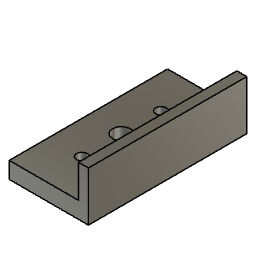
전방 덮개 브라켓 (Autodesk Fusion 360 design; units mm, degrees)
Autodesk Fusion 360 part; units mm, degrees
sketch "스케치1" plane through (0, 0, 0) normal (0, 0, 1) x (1, 0, 0)
  line L0 (10, 24) -> (-10, 24)
  line L1 (-10, 24) -> (-10, -24)
  line L2 (-10, -24) -> (10, -24)
  line L3 (10, -24) -> (10, 24)
  line L4 (10, 24) -> (-10, -24) construction
  line L5 (-10, 24) -> (10, -24) construction
  circle A0 centre (0, 0) radius 2.65
  line L6 (0, 0) -> (0, 12)
  circle A1 centre (0, 12) radius 1.6
  line L7 (0, 0) -> (0, -12)
  circle A2 centre (0, -12) radius 1.6
  line L8 (10, 24) -> (11, 24)
  line L9 (11, 24) -> (11, -24)
  line L10 (11, -24) -> (10, -24)
  line L11 (10, -24) -> (10, 24)
  line L12 (11, 24) -> (14, 24)
  line L13 (14, 24) -> (14, -24)
  line L14 (14, -24) -> (11, -24)
  line L15 (11, -24) -> (11, 24)
  line L16 (10, -6) -> (14, -6)
  dimension "d1" = 20
  dimension "d2" = 48
  dimension "d3" = 5.3
  dimension "d4" = 12
  dimension "d5" = 3.2
  dimension "d6" = 12
  dimension "d7" = 3.2
  dimension "d12" = 3
  constraint horizontal L0
  constraint perpendicular L0 L1
  constraint parallel L0 L2
  constraint parallel L1 L3
  constraint coincident L4 A0.centre
  constraint coincident L5 A0.centre
  constraint coincident A0.centre L6.start
  constraint vertical L6
  constraint coincident L6.end A1.centre
  constraint vertical L7
  constraint coincident L7.end A2.centre
  constraint horizontal L8
  constraint vertical L9
  constraint horizontal L10
  constraint vertical L11
  constraint horizontal L12
  constraint vertical L13
  constraint horizontal L14
  constraint vertical L15
  constraint coincident L11 L16.start
  constraint coincident L13 L16.end
  constraint perpendicular L13 L16
  measures "d1" distance of L1.end L2.end
  measures "d2" distance of L0.end L1.end
  measures "d3" diameter of A0
  measures "d4" distance of A0.centre L6.end
  measures "d5" diameter of A1
  measures "d6" distance of A0.centre L7.end
  measures "d7" diameter of A2
  measures "d12" distance of L8.end L12.end
extrude "돌출1" add sketch "스케치1" along normal blind 5 contours L0 L1 L2 L3 L11 | L3 L8 L9 L11 L15 L16 | L3 L9 L10 L11 L15 L16
extrude "돌출2" add sketch "스케치1" along normal blind 2.8 contours A1 | A2
extrude "돌출3" add sketch "스케치1" along normal blind 15 contours L9 L12 L13 L15 L16 | L9 L13 L14 L15 L16
